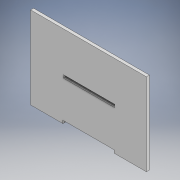
# Autodesk Inventor part: Frente
Saved by Autodesk Inventor 2020 (Build 240168000, 168)
## iProperties
Created: 2020-03-11
Part Number: Frente
Material: Generic
Document SubType Name: Modeling
Designer: José Javier Estrada
Density: 1 g/cm^3
Appearance: Default
Author: José Javier Estrada
Autodesk Inventor part; units mm, degrees
ref_plane "YZ Plane" through (0, 0, 0) normal (1, 0, 0) x (0, 1, 0)
ref_plane "XZ Plane" through (0, 0, 0) normal (0, 1, 0) x (-1, 0, 0)
ref_plane "XY Plane" through (0, 0, 0) normal (0, 0, 1) x (1, 0, 0)
sketch "Sketch1" plane through (0, 0, 0) normal (0, 0, 1) x (1, 0, 0)
  line L0 (0, 0) -> (-197, 0)
  line L1 (-197, 0) -> (-197, -140)
  line L2 (-197, -140) -> (0, -140)
  line L3 (0, -140) -> (0, 0)
  dimension "d0" = 140
  dimension "d1" = 197
  constraints: 8 end point, 2 parallel, 1 horizontal, 1 perpendicular
  measures "d0" distance of L0.end L1.end
  measures "d1" distance of L0.start L0.end
extrude "Extrusion1" add sketch "Sketch1" along normal blind 5
sketch "Sketch3" plane through (0, 0, 5) normal (0, 0, 1) x (1, 0, 0)
  line L0 (0, 0) -> (-197, 0) projected
  line L1 (0, -140) -> (0, 0) projected
  line L2 (-197, -140) -> (0, -140) projected
  line L3 (-197, 0) -> (-197, -140) projected
  line L4 (-142, -140) -> (-55, -140)
  line L5 (-55, -140) -> (-55, -135)
  line L6 (-55, -135) -> (-142, -135)
  line L7 (-142, -135) -> (-142, -140)
  line L8 (-141, -72.5) -> (-54, -72.5)
  line L9 (-54, -72.5) -> (-54, -67.5)
  line L10 (-54, -67.5) -> (-141, -67.5)
  line L11 (-141, -67.5) -> (-141, -72.5)
  point P0 (-55, -140)
  dimension "d13" = 5
  dimension "d14" = 55
  dimension "d15" = 55
  dimension "d16" = 5
  dimension "d17" = 72.5
  constraints: 16 end point, 4 parallel, 2 horizontal, 2 perpendicular, 1 collinear
  measures "d13" distance of L4.end L5.end
  measures "d14" distance between parallel lines of L1 L5
  measures "d15" distance between parallel lines of L3 L7
  measures "d16" distance of L8.end L9.end
  measures "d17" distance between parallel lines of L2 L10
extrude "Extrusion3" cut sketch "Sketch3" against normal blind 5 contours L2 L7 L6 L5 | L11 L10 L9 L8
body "Solid1"
